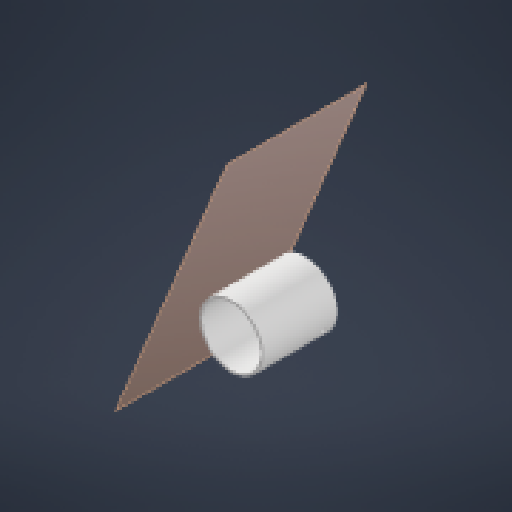
# Autodesk Inventor part: Part22
Saved by Autodesk Inventor 2027.1 (Build 311270010, 270A)
## iProperties
Created: 2026-09-29
Part Number: Part22
Material: Generic
Document SubType Name: Modeling
Designer: daniel
Density: 1 g/cm^3
Appearance: Default
Author: daniel
Autodesk Inventor part; units mm, degrees
ref_plane "YZ Plane" through (0, 0, 0) normal (1, 0, 0) x (0, 1, 0)
ref_plane "XZ Plane" through (0, 0, 0) normal (0, 1, 0) x (-1, 0, 0)
ref_plane "XY Plane" through (0, 0, 0) normal (0, 0, 1) x (1, 0, 0)
sketch "Sketch1" plane through (0, 0, 0) normal (0, 0, 1) x (1, 0, 0)
  circle A0 centre (0, 0) radius 27.5
  circle A1 centre (0, 0) radius 30
  dimension "d0" = 55
  dimension "d1" = 60
  constraints: 2 centre point, 2 coincident
  measures "d0" diameter of A0
  measures "d1" diameter of A1
extrude "Extrusion1" add sketch "Sketch1" along normal blind 70
ref_plane "Work Plane1" through (-98.6132, -98.2801, 30) normal (0.9239, -0.3827, 0) x (0.3827, 0.9239, 0)
ref_plane "Work Plane2" through (-98.6132, -98.2801, 30) normal (0.9239, -0.3827, 0) x (0.3827, 0.9239, 0)
sketch "Sketch2" plane through (-98.6132, -98.2801, 30) normal (0.9239, -0.3827, 0) x (0.3827, 0.9239, 0)
  circle A0 centre (128.5352, -20) radius 2.5
  line L0 (158.5352, -30) -> (98.5352, -30) projected
  point P0 (128.5352, -30)
  dimension "d4" = 5
  dimension "d5" = 10
  constraints: 1 centre point
  measures "d4" diameter of A0
  measures "d5" distance from line of L0 A0.centre
extrude "Extrusion2" cut sketch "Sketch2" along normal through all
equation "\"ProductBaseHeight\" = 35"
equation "\"GridProcutClearance\" = 3"
equation "\"GridBorderThickness\" = 5"
equation "\"GridBorderFillets\" = 7"
equation "\"GridTotalSize\" = 63"
equation "\"BaseTotalWidth\" = 352"
body "Solid1"
